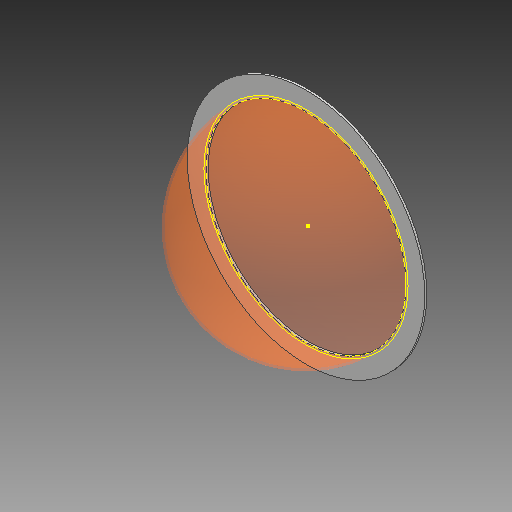
# Autodesk Inventor part: Futterschüssel_innen
Saved by Autodesk Inventor 2018 (Build 220112000, 112)
## iProperties
Created: 2017-09-29
Part Number: Futterschüssel_innen
Material: Generisch
Document SubType Name: Modeling
Designer: Dominik
Density: 1 g/cm^3
Appearance: Vorgabe
Mass: 2.96881 g
Surface Area: 65.9734 cm^2
Volume: 2.96881 cm^3
Author: Dominik
Autodesk Inventor part; units mm, degrees
ref_plane "YZ Plane" through (0, 0, 0) normal (1, 0, 0) x (0, 1, 0)
ref_plane "XZ Plane" through (0, 0, 0) normal (0, 1, 0) x (-1, 0, 0)
ref_plane "XY Plane" through (0, 0, 0) normal (0, 0, 1) x (1, 0, 0)
sketch "Skizze5" plane through (0, 0, 0) normal (0, 0, 1) x (1, 0, 0)
  line L0 (0, 0) -> (0, -48)
  arc A0 (-48, 0) -> (0, -48) centre (0, 0) ccw
  dimension "d17" = 48
  constraints: 2 end point, 2 point on circle, 1 centre point, 1 coincident, 1 vertical
  measures "d17" distance of L0.start L0.end
surface revolve "Rotationsfläche3" sketch "Skizze5" angle 360 about axis through (0, 0, 0) along (0, -1, 0) shown yes curves A0 L0
sketch "Skizze6" plane through (0, 0, 0) normal (0, 0, 1) x (1, 0, 0)
  line L0 (0, 0) -> (0, -49)
  arc A0 (-49, 0) -> (0, -49) centre (0, 0) ccw
  dimension "d19" = 49
  constraints: 2 end point, 2 point on circle, 1 centre point, 1 coincident, 1 vertical
  measures "d19" distance of L0.start L0.end
surface revolve "Rotationsfläche4" sketch "Skizze6" angle 360 about axis through (0, 0, 0) along (0, -1, 0) shown yes curves A0 L0
sketch "Skizze7" plane through (0, 0, 0) normal (0, 1, 0) x (-1, 0, 0)
  circle A0 centre (0, 0) radius 57
  dimension "d21" = 114
  constraints: 1 centre point, 1 coincident
  measures "d21" diameter of A0
extrude "Extrusion1" add sketch "Skizze7" along normal blind 1
sketch "Skizze8" plane through (0, 1, 0) normal (0, 1, 0) x (1, 0, 0)
  point P0 (0, 0)
sketch "Skizze9" plane through (0, 1, 0) normal (0, 1, 0) x (1, 0, 0)
  circle A0 centre (0, 0) radius 48
  constraints: 1 centre point, 1 coincident
extrude "Extrusion2" cut sketch "Skizze9" against normal blind 1
